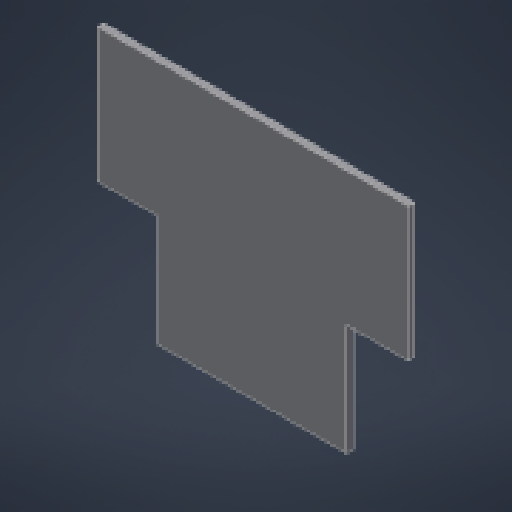
# Autodesk Inventor part: Dach
Saved by Autodesk Inventor 2023 (Build 270158000, 158)
## iProperties
Created: 2023-03-16
Part Number: Dach
Material: Generic
Document SubType Name: Modeling
Designer: Michał
Density: 1 g/cm^3
Appearance: Default
Author: Michał
Autodesk Inventor part; units mm, degrees
ref_plane "YZ Plane" through (0, 0, 0) normal (1, 0, 0) x (0, 1, 0)
ref_plane "XZ Plane" through (0, 0, 0) normal (0, 1, 0) x (-1, 0, 0)
ref_plane "XY Plane" through (0, 0, 0) normal (0, 0, 1) x (1, 0, 0)
sketch "Sketch1" plane through (0, 0, 0) normal (0, 0, 1) x (1, 0, 0)
  line L0 (60.55, -6.6) -> (60.55, -27.4477) construction
  line L1 (1.05, -39.5) -> (1.05, -9.5) construction
  line L2 (-18.1, 33.2115) -> (-18.1, -9.4) construction
  line L3 (79.9, -9.4) -> (79.9, 33.0115) construction
  line L4 (79.9, 33.0115) -> (-18.1, 33.0115) construction
  line L5 (79.9, -44.6) -> (-18.1, -44.6) construction
  line L6 (60.55, -44.4) -> (1.05, -44.4)
  line L7 (1.05, -44.4) -> (1.05, -9.4)
  line L8 (1.05, -9.4) -> (60.55, -9.4)
  line L9 (60.55, -9.4) -> (60.55, -44.4)
  line L10 (79.9, 32.8115) -> (-18.1, 32.8115)
  line L11 (-18.1, 32.8115) -> (-18.1, -9.4)
  line L12 (-18.1, -9.4) -> (79.9, -9.4)
  line L13 (79.9, -9.4) -> (79.9, 32.8115)
  line L14 (60.55, -9.4) -> (79.9, -9.4) construction
  point P0 (0, 0)
  point P1 (1.05, -9.4)
extrude "Extrusion1" add sketch "Sketch1" along normal blind 2
sketch "Sketch2" plane through (0, 0, 2) normal (0, 0, 1) x (1, 0, 0)
  line L0 (53.3804, -31.4) -> (8.2196, -31.4) construction
  line L1 (8.2196, -31.4) -> (8.2196, -23.7295) construction
  line L2 (8.2196, -23.7295) -> (53.3804, -23.7295) construction
  line L3 (53.3804, -23.7295) -> (53.3804, -31.4) construction
  line L4 (53.3804, -27.5648) -> (60.55, -27.5648) construction
  line L5 (60.55, -44.4) -> (60.55, -9.4) construction
  line L6 (8.2196, -27.5648) -> (1.05, -27.5648) construction
  line L7 (1.05, -9.4) -> (1.05, -44.4) construction
  line L8 (1.05, -44.4) -> (60.55, -44.4) construction
  line L9 (53.3804, -23.7295) -> (53.3804, -21.7295) construction
  line L10 (53.3804, -21.7295) -> (39.3804, -21.7295) construction
  line L11 (39.3804, -21.7295) -> (39.3804, -17.2295) construction
  line L12 (39.3804, -17.2295) -> (53.3804, -17.2295) construction
  line L13 (53.3804, -17.2295) -> (53.3804, -21.7295) construction
  line L14 (46.8626, -25.3881) -> (48.4081, -25.3881)
  line L15 (48.4081, -25.3881) -> (48.4081, -26.6411)
  line L16 (48.4081, -26.6411) -> (48.8785, -27.0996)
  line L17 (48.8785, -27.0996) -> (51.831, -27.0996)
  line L18 (51.831, -27.0996) -> (51.831, -25.3881)
  line L19 (51.831, -25.3881) -> (53.3765, -24.5028)
  line L20 (53.3765, -24.5028) -> (53.3765, -30.5028)
  line L21 (53.3765, -30.5028) -> (48.0287, -30.5028)
  line L22 (48.0287, -30.5028) -> (46.8626, -28.9336)
  line L23 (46.8626, -28.9336) -> (47.748, -27.7439)
  line L24 (47.748, -27.7439) -> (46.8626, -26.8545)
  line L25 (46.8626, -26.8545) -> (46.8626, -25.3881)
  line L26 (48.4516, -28.8269) -> (48.8626, -29.3644)
  line L27 (48.8626, -29.3644) -> (51.831, -29.3644)
  line L28 (51.831, -29.3644) -> (51.831, -28.2617)
  line L29 (51.831, -28.2617) -> (48.8666, -28.2617)
  line L30 (48.8666, -28.2617) -> (48.4516, -28.8269)
  line L31 (39.3923, -26.5502) -> (40.5543, -25.3881)
  line L32 (40.5543, -25.3881) -> (44.8231, -25.3881)
  line L33 (44.8231, -25.3881) -> (45.9852, -26.5502)
  line L34 (45.9852, -26.5502) -> (45.9852, -29.3407)
  line L35 (45.9852, -29.3407) -> (44.8231, -30.5028)
  line L36 (44.8231, -30.5028) -> (40.5543, -30.5028)
  line L37 (40.5543, -30.5028) -> (39.3923, -29.3407)
  line L38 (39.3923, -29.3407) -> (39.3923, -26.5502)
  line L39 (40.9377, -26.5265) -> (40.9377, -29.3644)
  line L40 (40.9377, -29.3644) -> (44.4397, -29.3644)
  line L41 (44.4397, -29.3644) -> (44.4397, -26.5265)
  line L42 (44.4397, -26.5265) -> (40.9377, -26.5265)
  line L43 (31.9852, -26.9534) -> (33.1472, -25.3802)
  line L44 (33.1472, -25.3802) -> (38.5662, -25.3802)
  line L45 (38.5662, -25.3802) -> (38.5662, -30.5028)
  line L46 (38.5662, -30.5028) -> (33.1472, -30.5028)
  line L47 (33.1472, -30.5028) -> (31.9852, -28.9296)
  line L48 (31.9852, -28.9296) -> (32.7124, -27.9415)
  line L49 (32.7124, -27.9415) -> (31.9852, -26.9534)
  line L50 (33.6769, -26.9534) -> (34.0524, -27.4198)
  line L51 (34.0524, -27.4198) -> (37.0207, -27.4198)
  line L52 (37.0207, -27.4198) -> (37.0207, -26.5265)
  line L53 (37.0207, -26.5265) -> (34.0524, -26.5265)
  line L54 (34.0524, -26.5265) -> (33.6769, -26.9534)
  line L55 (33.6769, -28.9296) -> (34.0524, -29.3565)
  line L56 (34.0524, -29.3565) -> (37.0207, -29.3565)
  line L57 (37.0207, -29.3565) -> (37.0207, -28.4632)
  line L58 (37.0207, -28.4632) -> (34.0524, -28.4632)
  line L59 (34.0524, -28.4632) -> (33.6769, -28.9296)
  line L60 (24.582, -26.5502) -> (25.7441, -25.3881)
  line L61 (25.7441, -25.3881) -> (30.0128, -25.3881)
  line L62 (30.0128, -25.3881) -> (31.1749, -26.5502)
  line L63 (31.1749, -26.5502) -> (31.1749, -29.3407)
  line L64 (31.1749, -29.3407) -> (30.0128, -30.5028)
  line L65 (30.0128, -30.5028) -> (25.7441, -30.5028)
  line L66 (25.7441, -30.5028) -> (24.582, -29.3407)
  line L67 (24.582, -29.3407) -> (24.582, -26.5502)
  line L68 (26.1275, -26.5265) -> (26.1275, -29.3644)
  line L69 (26.1275, -29.3644) -> (29.6294, -29.3644)
  line L70 (29.6294, -29.3644) -> (29.6294, -26.5265)
  line L71 (29.6294, -26.5265) -> (26.1275, -26.5265)
  line L72 (22.2105, -25.3802) -> (23.7559, -24.5028)
  line L73 (23.7559, -24.5028) -> (23.7559, -30.5028)
  line L74 (23.7559, -30.5028) -> (22.2105, -30.5028)
  line L75 (22.2105, -30.5028) -> (22.2105, -25.3802)
  line L76 (15.3923, -26.5265) -> (16.5385, -25.3802)
  line L77 (16.5385, -25.3802) -> (21.333, -25.3802)
  line L78 (21.333, -25.3802) -> (21.333, -30.5067)
  line L79 (21.333, -30.5067) -> (19.7875, -31.4)
  line L80 (19.7875, -31.4) -> (19.7875, -26.5265)
  line L81 (19.7875, -26.5265) -> (15.3923, -26.5265)
  line L82 (8.6255, -26.5502) -> (9.7875, -25.3881)
  line L83 (9.7875, -25.3881) -> (14.0563, -25.3881)
  line L84 (14.0563, -25.3881) -> (15.2184, -26.5502)
  line L85 (15.2184, -26.5502) -> (15.2184, -29.3407)
  line L86 (15.2184, -29.3407) -> (14.0563, -30.5028)
  line L87 (14.0563, -30.5028) -> (9.7875, -30.5028)
  line L88 (9.7875, -30.5028) -> (8.6255, -29.3407)
  line L89 (8.6255, -29.3407) -> (8.6255, -26.5502)
  line L90 (10.1709, -26.5265) -> (10.1709, -29.3644)
  line L91 (10.1709, -29.3644) -> (13.6729, -29.3644)
  line L92 (13.6729, -29.3644) -> (13.6729, -26.5265)
  line L93 (13.6729, -26.5265) -> (10.1709, -26.5265)
  line L94 (48.6426, -19.3685) -> (49.4173, -18.3198)
  line L95 (49.4173, -18.3198) -> (53.3778, -18.3198)
  line L96 (53.3778, -18.3198) -> (52.6189, -19.0786)
  line L97 (52.6189, -19.0786) -> (50.0207, -19.0786)
  line L98 (50.0207, -19.0786) -> (49.7783, -19.3685)
  line L99 (49.7783, -19.3685) -> (50.0181, -19.6742)
  line L100 (50.0181, -19.6742) -> (52.6242, -19.6742)
  line L101 (52.6242, -19.6742) -> (53.3778, -20.6808)
  line L102 (53.3778, -20.6808) -> (52.6031, -21.7295)
  line L103 (52.6031, -21.7295) -> (48.6426, -21.7295)
  line L104 (48.6426, -21.7295) -> (49.4068, -20.9706)
  line L105 (49.4068, -20.9706) -> (51.9997, -20.9706)
  line L106 (51.9997, -20.9706) -> (52.25, -20.6808)
  line L107 (52.25, -20.6808) -> (51.9997, -20.3751)
  line L108 (51.9997, -20.3751) -> (49.3936, -20.3751)
  line L109 (49.3936, -20.3751) -> (48.6426, -19.3685)
  line L110 (44.1314, -21.7295) -> (44.8903, -20.9653)
  line L111 (44.8903, -20.9653) -> (47.1828, -20.9653)
  line L112 (47.1828, -20.9653) -> (47.1828, -20.3698)
  line L113 (47.1828, -20.3698) -> (44.6294, -20.3698)
  line L114 (44.6294, -20.3698) -> (45.3251, -19.6742)
  line L115 (45.3251, -19.6742) -> (47.1828, -19.6742)
  line L116 (47.1828, -19.6742) -> (47.1828, -19.0786)
  line L117 (47.1828, -19.0786) -> (44.2526, -19.0786)
  line L118 (44.2526, -19.0786) -> (45.0168, -18.3145)
  line L119 (45.0168, -18.3145) -> (48.2131, -18.3145)
  line L120 (48.2131, -18.3145) -> (48.2131, -21.7295)
  line L121 (48.2131, -21.7295) -> (44.1314, -21.7295)
  line L122 (39.4516, -18.3198) -> (40.4819, -18.3198)
  line L123 (40.4819, -18.3198) -> (40.4819, -19.1551)
  line L124 (40.4819, -19.1551) -> (40.7954, -19.4607)
  line L125 (40.7954, -19.4607) -> (42.7638, -19.4607)
  line L126 (42.7638, -19.4607) -> (42.7638, -18.3198)
  line L127 (42.7638, -18.3198) -> (43.7941, -17.7295)
  line L128 (43.7941, -17.7295) -> (43.7941, -21.7295)
  line L129 (43.7941, -21.7295) -> (40.2289, -21.7295)
  line L130 (40.2289, -21.7295) -> (39.4516, -20.6834)
  line L131 (39.4516, -20.6834) -> (40.0418, -19.8902)
  line L132 (40.0418, -19.8902) -> (39.4516, -19.2974)
  line L133 (39.4516, -19.2974) -> (39.4516, -18.3198)
  line L134 (40.5109, -20.6122) -> (40.7849, -20.9706)
  line L135 (40.7849, -20.9706) -> (42.7638, -20.9706)
  line L136 (42.7638, -20.9706) -> (42.7638, -20.2354)
  line L137 (42.7638, -20.2354) -> (40.7875, -20.2354)
  line L138 (40.7875, -20.2354) -> (40.5109, -20.6122)
  point P0 (0, 0)
  dimension "d0" = 0.2
  dimension "d1" = 0.2
  dimension "d4" = 13
  dimension "d5" = 2
  dimension "d6" = 7.6705
  dimension "d7" = 45.1609
  dimension "d8" = 4.5
  dimension "d9" = 14
  constraints: 6 end point, 3 point on line, 2 collinear, 2 horizontal, 2 midpoint, 1 coincident, 1 vertical, 4 other
  measures "d4" distance between parallel lines of L8 L0
  measures "d5" distance of L2.end L9.end
  measures "d6" distance between parallel lines of L0 L2
  measures "d7" distance between parallel lines of L1 L3
  measures "d8" distance between parallel lines of L10 L12
  measures "d9" distance between parallel lines of L11 L13
extrude "Extrusion2" cut sketch "Sketch2" against normal blind 1
sketch "Sketch3" plane through (0, 0, 2) normal (0, 0, 1) x (1, 0, 0)
  circle A0 centre (-15.6, 3.6) radius 1.2295 projected
  arc A1 (76.247, 4.027) -> (76.9, 4.7232) centre (77.4, 3.6) ccw projected
  point P0 (0, 0)
hole "Hole1" at (77.4, 3.6, 2) at (-15.6, 3.6, 2) direction (0, 0, -1) diameter 3.4 end through all countersink diameter 6.3 countersink angle 90 clearance for "Countersunk Flat Head Screw ISO 2009/7046" size "M3" standard "ISO"
body "Solid1"
